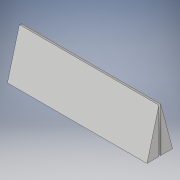
# Autodesk Inventor part: sideFoldSupport
Saved by Autodesk Inventor 2019 (Build 230136000, 136)
## iProperties
Created: 2018-07-17
Part Number: sideFoldSupport
Material: Generic
Document SubType Name: Modeling
Designer: Ge Shi
Density: 1 g/cm^3
Appearance: Default
Author: Ge Shi
Autodesk Inventor part; units mm, degrees
ref_plane "YZ Plane" through (0, 0, 0) normal (1, 0, 0) x (0, 1, 0)
ref_plane "XZ Plane" through (0, 0, 0) normal (0, 1, 0) x (-1, 0, 0)
ref_plane "XY Plane" through (0, 0, 0) normal (0, 0, 1) x (1, 0, 0)
sketch "Sketch1" plane through (0, 0, 0) normal (1, 0, 0) x (0, 1, 0)
  line L0 (0, 0.7604) -> (39.9222, 0.7604)
  line L1 (39.9222, 0.7604) -> (0, 11.4575)
  line L2 (0, -11.4575) -> (40, -0.7396)
  line L3 (40, -0.7396) -> (0, -0.7396)
  line L4 (0, 0) -> (3.0655, 0) construction
  line L5 (0, 11.4575) -> (0, 0.7604)
  line L6 (0, -0.7396) -> (0, -11.4575)
  dimension "d0" = 1.5
  dimension "d2" = 15
  constraints: 14 end point, 1 collinear, 1 horizontal, 1 parallel, 1 vertical, 1 other
  measures "d0" distance between parallel lines of L0 L3
  measures "d2" angle of L1 L0
extrude "Extrusion1" add sketch "Sketch1" along normal blind 125
equation "\"d0\" = thickness"
equation "\"d3\" = 5 * width"
equation "\"thickness\" = 1.5"
equation "\"width\" = 25"
body "Solid1"
